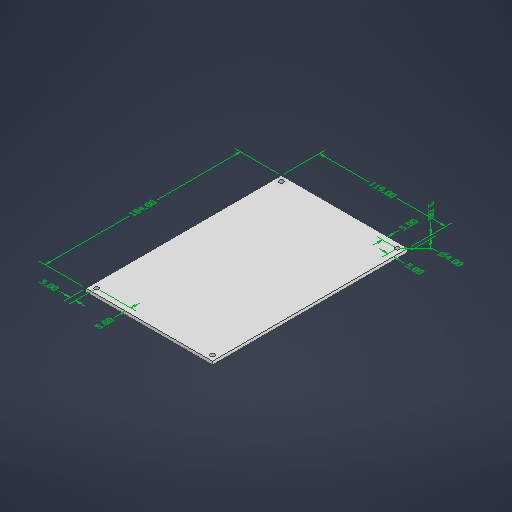
# Autodesk Inventor part: RobotBreadBoardBoard
Saved by Autodesk Inventor 2026 (Build 300175000, 175)
## iProperties
Created: 2025-07-21
Part Number: RobotBreadBoardBoard
Material: Generic
Document SubType Name: Modeling
Designer: jsmal
Density: 1 g/cm^3
Appearance: Default
Author: jsmal
Autodesk Inventor part; units mm, degrees
ref_plane "YZ Plane" through (0, 0, 0) normal (1, 0, 0) x (0, 1, 0)
ref_plane "XZ Plane" through (0, 0, 0) normal (0, 1, 0) x (-1, 0, 0)
ref_plane "XY Plane" through (0, 0, 0) normal (0, 0, 1) x (1, 0, 0)
sketch "Sketch1" plane through (0, 0, 0) normal (0, 1, 0) x (-1, 0, 0)
  line L0 (0, 0) -> (119, 0)
  line L1 (119, 0) -> (119, -184)
  line L2 (119, -184) -> (0, -184)
  line L3 (0, -184) -> (0, 0)
  dimension "d0" = 119
  dimension "d1" = 184
  constraints: 8 end point, 2 parallel, 1 horizontal, 1 perpendicular
  measures "d0" distance of L1.end L2.end
  measures "d1" distance of L0.end L1.end
extrude "Extrusion1" add sketch "Sketch1" along normal blind 3
sketch "Sketch2" plane through (0, 3, 0) normal (0, 1, 0) x (1, 0, 0)
  circle A0 centre (-114, 5) radius 2
  line L0 (-119, 184) -> (-119, 0) projected
  line L1 (-119, 0) -> (0, 0) projected
  circle A1 centre (-114, 179) radius 2
  line L2 (0, 184) -> (-119, 184) projected
  circle A2 centre (-5, 179) radius 2
  line L3 (0, 0) -> (0, 184) projected
  circle A3 centre (-5, 5) radius 2
  dimension "d4" = 4
  dimension "d5" = 5
  dimension "d6" = 5
  dimension "d7" = 4
  dimension "d8" = 5
  dimension "d9" = 5
  dimension "d10" = 4
  dimension "d11" = 5
  dimension "d12" = 5
  dimension "d13" = 4
  dimension "d14" = 5
  dimension "d15" = 5
  constraints: 4 centre point
  measures "d4" diameter of A0
  measures "d5" distance from line of L0 A0.centre
  measures "d6" distance from line of A0.centre L1
  measures "d7" diameter of A1
  measures "d8" distance from line of L0 A1.centre
  measures "d9" distance from line of L2 A1.centre
  measures "d10" diameter of A2
  measures "d11" distance from line of L3 A2.centre
  measures "d12" distance from line of L2 A2.centre
  measures "d13" diameter of A3
  measures "d14" distance from line of L1 A3.centre
  measures "d15" distance from line of L3 A3.centre
extrude "Extrusion2" cut sketch "Sketch2" against normal blind 3 contours A0 | A1 | A2 | A3
body "Solid1"
